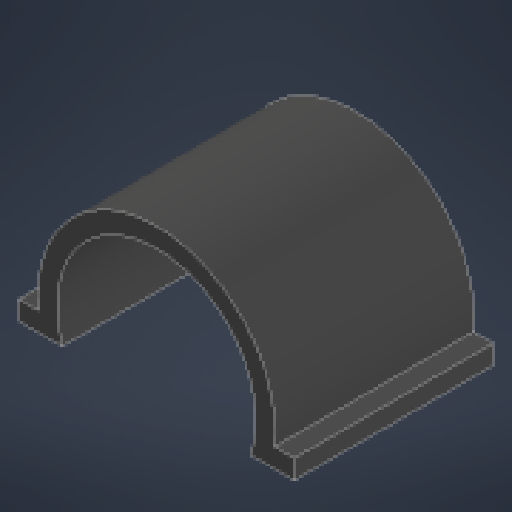
# Autodesk Inventor part: rotion_stopper
Saved by Autodesk Inventor 2026.1 (Build 301233020, 233B)
## iProperties
Created: 2025-12-02
Part Number: rotion_stopper
Material: 고무, 검은색
Document SubType Name: Modeling
Designer: jaewook
Density: 0.93 g/cm^3
Appearance: 고무 - 검은색
Author: jaewook
Autodesk Inventor part; units mm, degrees
ref_plane "YZ Plane" through (0, 0, 0) normal (1, 0, 0) x (0, 1, 0)
ref_plane "XZ Plane" through (0, 0, 0) normal (0, 1, 0) x (-1, 0, 0)
ref_plane "XY Plane" through (0, 0, 0) normal (0, 0, 1) x (1, 0, 0)
sketch "스케치1" plane through (0, 0, 0) normal (0, 0, 1) x (1, 0, 0)
  arc A0 (4.9143, -1.7) -> (-4.9143, -1.7) centre (0, 0) ccw
  line L0 (-7.2, -1.7) -> (-7.2, -0.7)
  line L1 (7.2, -0.7) -> (7.2, -1.7)
  arc A1 (5.9624, -1.7) -> (-6.1604, -0.7) centre (0, 0) ccw
  line L2 (-7.2, -1.7) -> (-4.9143, -1.7)
  line L3 (4.9143, -1.7) -> (7.2, -1.7)
  line L4 (-7.2, -0.7) -> (-5.1527, -0.7)
  line L5 (5.1527, -0.7) -> (7.2, -0.7)
  point P0 (0, -0.7)
  point P1 (6.1604, -0.7)
  dimension "d0" = 10.4
  dimension "d1" = 1
  dimension "d2" = 0.7
  dimension "d3" = 2
  dimension "d4" = 1
  constraints: 12 end point, 6 point on circle, 4 perpendicular, 3 collinear, 2 centre point, 2 horizontal, 2 point on line, 1 coincident, 1 horizontal alignment, 1 vertical, 1 vertical alignment
  measures "d0" diameter of A0
  measures "d1" distance of L0.start L0.end
  measures "d2" distance of point (0, 0) point (0, -0.7)
  measures "d3" distance edge to line of A0 L0
  measures "d4" radial gap between concentric circles of A0 A1
extrude "돌출1" add sketch "스케치1" along normal blind 10.4
